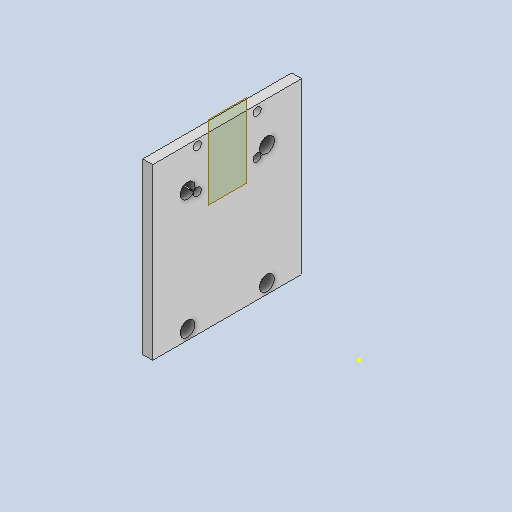
# Autodesk Inventor part: соединяет крепление с магнитом и рельсу
Saved by Autodesk Inventor 2024.2 (Build 282272000, 272)
## iProperties
Created: 2026-01-31
Part Number: соединяет крепление с магнитом и рельсу
Material: Типовые
Document SubType Name: Modeling
Designer: katya_notebook
Density: 1 g/cm^3
Appearance: По умолчанию
Author: katya_notebook
Autodesk Inventor part; units mm, degrees
ref_plane "YZ Plane" through (0, 0, 0) normal (1, 0, 0) x (0, 1, 0)
ref_plane "XZ Plane" through (0, 0, 0) normal (0, 1, 0) x (-1, 0, 0)
ref_plane "XY Plane" through (0, 0, 0) normal (0, 0, 1) x (1, 0, 0)
ref_plane "РабПлоскость1" through (-25.9085, 44.7403, 28.4958) normal (-1, 0, 0) x (0, 0, -1)
sketch "Эскиз1" plane through (-25.9085, 44.7403, 28.4958) normal (-1, 0, 0) x (0, 0, -1)
  circle A0 centre (6, -10.75) radius 1.2 projected
  circle A1 centre (6, -2.75) radius 1.2 projected
  circle A2 centre (-6, -2.75) radius 1.2 projected
  circle A3 centre (-6, -10.75) radius 0.8 projected
  circle A4 centre (6, -10.75) radius 0.8 projected
  circle A5 centre (6, -2.75) radius 0.8 projected
  circle A6 centre (-6, -2.75) radius 0.8 projected
  line L0 (6, -10.75) -> (0, -10.75)
  line L1 (0, -10.75) -> (0, 50.15)
  line L2 (-14.95, 8.05) -> (14.95, 8.05)
  line L3 (14.95, 8.05) -> (14.95, -11.95)
  line L4 (14.95, -11.95) -> (-14.95, -11.95)
  line L5 (-14.95, -11.95) -> (-14.95, 8.05)
  line L6 (-14.95, 8.05) -> (14.95, -11.95) construction
  line L7 (14.95, 8.05) -> (-14.95, -11.95) construction
  line L8 (-8.0537, -1.95) -> (-31.9537, -1.95) projected
  point P0 (28.4958, 44.7403)
  point P1 (0, -1.95)
  dimension "d0" = 6
  dimension "d1" = 29.9
  dimension "d2" = 20
  constraints: 16 end point, 2 horizontal, 2 midpoint, 2 parallel, 2 point on line, 1 perpendicular, 1 vertical
  measures "d0" distance of L0.start L0.end
  measures "d1" distance of L3.end L4.end
  measures "d2" distance of L2.end L3.end
extrude "Выдавливание1" add sketch "Эскиз1" along normal blind 2 contours A0 | A0 L0 L1 L2 L3 L4 | A0 L4 L5 L2 L1 L0 | A1 | A2
sketch "Эскиз2" plane through (-27.9085, 44.7403, 28.4958) normal (-1, 0, 0) x (0, 0, 1)
  line L0 (-14.95, 11.95) -> (-14.95, -8.05) projected
  line L1 (-14.95, -8.05) -> (14.95, -8.05)
  line L2 (14.95, -8.05) -> (14.95, -22.05)
  line L3 (14.95, -22.05) -> (-14.95, -22.05)
  line L4 (-14.95, -22.05) -> (-14.95, -8.05)
  point P0 (-28.4958, -44.7403)
  dimension "d5" = 14
  constraints: 8 end point, 2 parallel, 1 horizontal, 1 perpendicular
  measures "d5" distance of L1.end L2.end
extrude "Выдавливание2" add sketch "Эскиз2" against normal blind 2
sketch "Эскиз3" plane through (-27.9085, 44.7403, 28.4958) normal (-1, 0, 0) x (0, 0, 1)
  point P0 (-28.4958, -44.7403)
sketch "Эскиз4" plane through (-27.9085, 44.7403, 28.4958) normal (-1, 0, 0) x (0, 0, 1)
  circle A0 centre (-7.95, 3.95) radius 1.5 projected
  circle A1 centre (-7.95, -20.05) radius 1.5 projected
  circle A2 centre (7.95, -20.05) radius 1.5 projected
  circle A3 centre (7.95, 3.95) radius 1.5 projected
  point P0 (-28.4958, -44.7403)
extrude "Выдавливание3" cut sketch "Эскиз4" against normal blind 2
